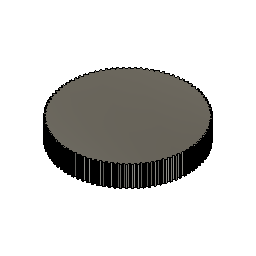
gear_90z (Autodesk Fusion 360 design; units mm, degrees)
Autodesk Fusion 360 part; units mm, degrees
sketch "Sketch1" plane through (0, 0, 0) normal (0, 0, 1) x (1, 0, 0) in component "gt2 pulley"
  circle A0 centre (0, 0) radius 28.6479 construction
  circle A1 centre (0, 0) radius 27.6439 construction
  line L0 (0, 0) -> (0, 28.6479) construction
  line L1 (0, 0) -> (0.9998, 28.6304) construction
  line L2 (0, 0) -> (1.4044, 28.6134) construction
  circle A2 centre (0, 0) radius 28.3939 construction
  arc A3 (0.3971, 28.2581) -> (0.4755, 27.9597) centre (1.392, 28.3598) ccw
  circle A4 centre (0, 0) radius 28.2439 construction
  arc A5 (0.2492, 28.3928) -> (0, 28.3939) centre (0, 0) ccw
  arc A6 (0.3971, 28.2581) -> (0.2492, 28.3928) centre (0.2479, 28.2428) ccw
  arc A7 (0.4755, 27.9597) -> (0.9648, 27.627) centre (0.9841, 28.1817) ccw
  arc A8 (0, 28.3939) -> (-0.2492, 28.3928) centre (0, 0) ccw
  arc A9 (-0.2492, 28.3928) -> (-0.3971, 28.2581) centre (-0.2479, 28.2428) ccw
  arc A10 (-0.4755, 27.9597) -> (-0.3971, 28.2581) centre (-1.392, 28.3598) ccw
  arc A11 (-0.9649, 27.627) -> (-0.4755, 27.9597) centre (-0.9841, 28.1817) ccw
  arc A12 (0.9648, 27.627) -> (-0.9648, 27.627) centre (0, 0) ccw
  point P0 (1.392, 28.3598)
  point P1 (0, 28.3939)
  dimension "d18" = 57.2958
  dimension "d19" = 2
  dimension "d22" = 1.004
  dimension "d24" = 0.75
  dimension "d26" = 1
  dimension "d27" = 0.15
  dimension "d28" = 0.15
  dimension "d47" = 0.555
  dimension "d52" = 3.812
  constraint coincident A0.centre A1.centre
  constraint coincident A0 L0.end
  constraint vertical L0
  constraint coincident A0 L1.end
  constraint coincident A0 L2.end
  constraint concentric A1 A2
  constraint coincident A1 A7.end
  constraint coincident L1 A7.end
  constraint coincident A2 P0
  constraint coincident L2 P0
  constraint coincident P0 A3.centre
  constraint coincident A2 P1
  constraint coincident L0 P1
  constraint concentric A2 A4
  constraint coincident P1 A5.end
  constraint coincident A4 A6.centre
  constraint coincident A3.start A6.start
  constraint tangent A3 A6
  constraint tangent A3 A7
  constraint symmetric L0 A7.end A12.end
  constraint symmetric L0 A3.start A9.end
  constraint symmetric L0 A3.end A10.start
  constraint symmetric L0 A3 A10
  constraint symmetric L0 A5.start A8.end
  constraint symmetric L0 P1 A5.end
  constraint symmetric L0 A5 A8
  constraint symmetric L0 A6 A9
  constraint symmetric L0 A7 A11
  constraint coincident A1 A11.start
  constraint tangent A1 A7
  constraint coincident L1 A7.centre
  measures "d18" diameter of A0
  measures "d19" angle of L0 L1
  measures "d22" distance of A0 A1
  measures "d24" distance of A1 A2
  measures "d26" radius of A3
  measures "d27" distance of A2 A4
  measures "d28" radius of A6
  measures "d47" radius of A7
extrude "Extrude1" add sketch "Sketch1" along normal blind 10 makes body 1
pattern_circular "C-Pattern1" count 90 over 360 about axis through (0, 0, 1.75) along (0, 0, 1) of bodies 1 makes body 2 at (-1.179, 27.6187, 3.3333) makes body 3 at (-3.9535, 27.3597, 6.6667) makes body 4 at (-6.4795, 26.8738, 6.6667) makes body 5 at (-6.8955, 26.7701, 3.3333) makes body 6 at (-9.5555, 25.9399, 6.6667) makes body 7 at (-11.9253, 24.9394, 6.6667) makes body 8 at (-13.6359, 24.0468, 6.6667) makes body 9 at (-15.2801, 23.037, 6.6667) makes body 10 at (-16.3353, 22.3012, 6.6667) makes body 11 at (-17.1877, 21.651, 3.3333) makes body 12 at (-18.6562, 20.3993, 3.3333) makes body 13 at (-21.038, 17.9328, 6.6667) makes body 14 at (-21.7175, 17.1036, 6.6667) makes body 15 at (-23.2133, 15.0109, 6.6667) makes body 16 at (-23.5563, 14.4667, 3.3333) makes body 17 at (-24.893, 12.0218, 6.6667) makes body 18 at (-25.9027, 9.6559, 6.6667) makes body 19 at (-26.3239, 8.4403, 6.6667) makes body 20 at (-26.8485, 6.5835, 6.6667) makes body 21 at (-27.3442, 4.0594, 6.6667) makes body 22 at (-27.4039, 3.6348, 6.6667) makes body 23 at (-27.6406, 0.4288, 6.6667) makes body 24 at (-27.6431, -0.2144, 3.3333) makes body 25 at (-27.481, -2.9962, 6.6667) makes body 26 at (-27.3442, -4.0595, 3.3333) makes body 27 at (-26.9944, -5.9571, 6.6667) makes body 28 at (-26.3238, -8.4404, 6.6667) makes body 29 at (-25.9026, -9.656, 3.3333) makes body 30 at (-25.166, -11.4393, 6.6667) makes body 31 at (-23.5562, -14.4668, 6.6667) makes body 32 at (-22.8577, -15.5471, 6.6667) makes body 33 at (-22.2377, -16.4217, 3.3333) makes body 34 at (-20.0336, -19.0483, 6.6667) makes body 35 at (-19.7358, -19.3567, 3.3333) makes body 36 at (-17.1877, -21.6511, 6.6667) makes body 37 at (-15.6355, -22.7973, 6.6667) makes body 38 at (-14.0072, -23.8324, 6.6667) makes body 39 at (-12.8832, -24.4583, 6.6667) makes body 40 at (-11.9252, -24.9394, 3.3333) makes body 41 at (-9.3539, -26.0133, 6.6667) makes body 42 at (-7.1029, -26.7158, 6.6667) makes body 43 at (-5.6425, -27.0619, 6.6667) makes body 44 at (-4.589, -27.2603, 6.6667) makes body 45 at (-1.1789, -27.6187, 6.6667) makes body 46 at (0.7505, -27.6337, 6.6667) makes body 47 at (2.4628, -27.534, 6.6667) makes body 48 at (4.5891, -27.2603, 6.6667) makes body 49 at (5.8524, -27.0173, 6.6667) makes body 50 at (6.8955, -26.7701, 3.3333) makes body 51 at (8.7461, -26.2238, 3.3333) makes body 52 at (11.9253, -24.9394, 6.6667) makes body 53 at (13.6359, -24.0468, 6.6667) makes body 54 at (14.7399, -23.3863, 6.6667) makes body 55 at (15.6356, -22.7972, 3.3333) makes body 56 at (17.1877, -21.651, 3.3333) makes body 57 at (19.2801, -19.8107, 6.6667) makes body 58 at (21.038, -17.9328, 6.6667) makes body 59 at (21.7175, -17.1036, 6.6667) makes body 60 at (23.3291, -14.8304, 6.6667) makes body 61 at (24.3067, -13.1669, 6.6667) makes body 62 at (24.508, -12.7883, 3.3333) makes body 63 at (25.671, -10.256, 6.6667) makes body 64 at (26.3239, -8.4403, 6.6667) makes body 65 at (26.8485, -6.5835, 6.6667) makes body 66 at (27.0836, -5.5376, 3.3333) makes body 67 at (27.5035, -2.7829, 6.6667) makes body 68 at (27.6406, -0.4288, 6.6667) makes body 69 at (27.6431, 0.2144, 3.3333) makes body 70 at (27.481, 2.9962, 6.6667) makes body 71 at (27.3442, 4.0595, 3.3333) makes body 72 at (26.6313, 7.4134, 6.6667) makes body 73 at (26.0493, 9.2531, 6.6667) makes body 74 at (25.9026, 9.656, 3.3333) makes body 75 at (25.166, 11.4393, 3.3333) makes body 76 at (23.5562, 14.4668, 6.6667) makes body 77 at (22.6137, 15.8998, 6.6667) makes body 78 at (21.3136, 17.6044, 6.6667) makes body 79 at (20.4715, 18.577, 6.6667) makes body 80 at (19.7358, 19.3567, 3.3333) makes body 81 at (17.1877, 21.6511, 6.6667) makes body 82 at (15.6355, 22.7973, 6.6667) makes body 83 at (14.0072, 23.8324, 6.6667) makes body 84 at (12.8832, 24.4583, 6.6667) makes body 85 at (11.9252, 24.9394, 3.3333) makes body 86 at (9.3539, 26.0133, 6.6667) makes body 87 at (8.3382, 26.3564, 3.3333) makes body 88 at (5.6425, 27.0619, 6.6667) makes body 89 at (3.9534, 27.3597, 6.6667) makes body 90 at (1.1789, 27.6187, 6.6667)
sketch "Sketch2" plane through (0, 0, 10) normal (0, 0, 1) x (-1, 0, 0)
  arc A0 (-15.3113, -23.7537) -> (-15.2572, -23.9464) centre (-15.1767, -23.8199) ccw
  arc A1 (-15.2572, -23.9464) -> (-14.8346, -24.2105) centre (0, 0) ccw
  arc A2 (-14.8346, -24.2105) -> (-14.6377, -24.1746) centre (-14.7562, -24.0826) ccw
  arc A3 (-14.4131, -23.9631) -> (-14.6377, -24.1746) centre (-13.8479, -24.7881) ccw
  arc A4 (-13.8219, -23.9403) -> (-14.4131, -23.9631) centre (-14.0994, -24.421) ccw
  arc A5 (-15.4583, -22.9178) -> (-13.8219, -23.9403) centre (0, 0) ccw
  arc A6 (-15.2196, -23.4592) -> (-15.4583, -22.9178) centre (-15.7686, -23.3779) ccw
  arc A7 (-15.3113, -23.7537) -> (-15.2196, -23.4592) centre (-16.2088, -23.3128) ccw
  circle A8 centre (0, 0) radius 27.6439
  constraint concentric A1 A8
extrude "Extrude2" add sketch "Sketch2" against normal blind 10 contours A5 A8 bodies 1 2 3 4 5 6 7 8 9 10 11 12 13 14 15 16 17 18 19 20 21 22 23 24 25 26 27 28 29 30 31 32 33 34 35 36 37 38 39 40 41 42 43 44 45 46 47 48 49 50 51 52 53 54 55 56 57 58 59 60 61 62 63 64 65 66 67 68 69 70 71 72 73 74 75 76 77 78 79 80 81 82 83 84 85 86 87 88 89 90
extrude "Extrude4" [suppressed] in component "gt2 pulley"
pattern_circular "C-Pattern7" [suppressed] in component "gt2 pulley"
extrude "Extrude3" [suppressed] in component "gt2 pulley"
pattern_circular "C-Pattern6" [suppressed] in component "gt2 pulley"
extrude "Extrude2'" [suppressed] in component "gt2 pulley"
pattern_circular "C-Pattern5" [suppressed] in component "gt2 pulley"
extrude "Extrude1'" [suppressed] in component "gt2 pulley"
pattern_circular "C-Pattern4" [suppressed] in component "gt2 pulley"
pattern_circular "C-Pattern3" [suppressed] in component "gt2 pulley"
pattern_circular "C-Pattern2" [suppressed] in component "gt2 pulley"
pattern_circular "C-Pattern1'" [suppressed] in component "gt2 pulley"
copy_body "Body->Comp1" [suppressed] in component "Component"
copy_body "Body->Comp2" [suppressed] in component "Component'"
copy_body "Body->Comp3" [suppressed] in component "Component''"
copy_body "Body->Comp4" [suppressed] in component "Component'''"
copy_body "Body->Comp5" [suppressed] in component "Component''''"
copy_body "Body->Comp6" [suppressed] in component "Component'''''"
copy_body "Body->Comp7" [suppressed] in component "Component''''''"
copy_body "Body->Comp8" [suppressed] in component "Component'''''''"
copy_body "Body->Comp9" [suppressed] in component "Component''''''''"
copy_body "Body->Comp10" [suppressed] in component "Component'''''''''"
copy_body "Body->Comp11" [suppressed] in component "Component''''''''''"
copy_body "Body->Comp12" [suppressed] in component "Component'''''''''''"
copy_body "Body->Comp13" [suppressed] in component "Component''''''''''''"
copy_body "Body->Comp14" [suppressed] in component "Component'''''''''''''"
copy_body "Body->Comp15" [suppressed] in component "Component''''''''''''''"
copy_body "Body->Comp16" [suppressed] in component "Component'''''''''''''''"
copy_body "Body->Comp17" [suppressed] in component "Component''''''''''''''''"
copy_body "Body->Comp18" [suppressed] in component "Component'''''''''''''''''"
copy_body "Body->Comp19" [suppressed] in component "Component''''''''''''''''''"
copy_body "Body->Comp20" [suppressed] in component "Component'''''''''''''''''''"
component "gt2 pulley" placed x (1, 0, 0) y (0, 1, 0) z (0, 0, 1) at (0, 0, 0)
equation "NumTeeth = 90" comment "min 20"
equation "ToothPitch = 2 mm"
equation "PullyDia = NumTeeth * ToothPitch / PI"
equation "ToothAng = ( ( 360 / NumTeeth ) * 1 deg )"
equation "TransOffsetAngle = ToothAng * 0.2"
equation "Sholulder_Radius = 0.15 mm"
equation "Root_Radius = 0.555 mm"
equation "TransRadius = 1 mm"
equation "ToolHeight = 0.75 mm"
equation "PLD = 0.254 mm"
equation "d18 = PullyDia"
equation "d19 = ToothAng / 2"
equation "d22 = PLD + ToolHeight"
equation "d24 = ToolHeight"
equation "d26 = TransRadius"
equation "d27 = Sholulder_Radius"
equation "d31 = NumTeeth"
equation "d33 = NumTeeth"
equation "d35 = NumTeeth"
equation "d37 = NumTeeth"
equation "d41 = NumTeeth"
equation "d45 = NumTeeth"
equation "d47 = Root_Radius"
equation "d50 = NumTeeth"
